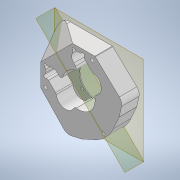
# Autodesk Inventor part: upper
Saved by Autodesk Inventor 2022 (Build 260153000, 153)
## iProperties
Created: 2022-03-17
Part Number: upper
Material: Generic
Document SubType Name: Modeling
Designer: zac-h
Density: 1 g/cm^3
Appearance: Default
Author: zac-h
Autodesk Inventor part; units mm, degrees
ref_plane "YZ Plane" through (0, 0, 0) normal (1, 0, 0) x (0, 1, 0)
ref_plane "XZ Plane" through (0, 0, 0) normal (0, 1, 0) x (-1, 0, 0)
ref_plane "XY Plane" through (0, 0, 0) normal (0, 0, 1) x (1, 0, 0)
ref_plane "Work Plane1" through (0, 0, 0) normal (0, 0, 1) x (1, 0, 0)
sketch "Sketch1" plane through (0, 0, 0) normal (0, 0, 1) x (1, 0, 0)
  line L0 (54.6745, 14.0094) -> (51.6007, 0.0667) projected
  arc A0 (54.6745, 14.0094) -> (51.7087, 23.6992) centre (44.6112, 16.228) ccw projected
  line L1 (19.1376, 54.6412) -> (51.7087, 23.6992) projected
  arc A1 (19.1376, 54.6412) -> (18.4488, 54.9162) centre (18.4488, 53.9162) ccw projected
  line L2 (-38.4967, 54.9162) -> (18.4488, 54.9162) projected
  arc A2 (-38.4967, 54.9162) -> (-54.9162, 38.4967) centre (-38.4967, 38.4967) ccw projected
  line L3 (-54.9162, -18.4488) -> (-54.9162, 38.4967) projected
  arc A3 (-54.9162, -18.4488) -> (-54.6412, -19.1376) centre (-53.9162, -18.4488) ccw projected
  line L4 (-23.6992, -51.7087) -> (-54.6412, -19.1376) projected
  arc A4 (-23.6992, -51.7087) -> (-14.0094, -54.6745) centre (-16.228, -44.6112) ccw projected
  line L5 (-0.0667, -51.6007) -> (-14.0094, -54.6745) projected
  arc A5 (-0.0667, -51.6007) -> (0.1266, -51.5369) centre (-0.282, -50.6241) ccw projected
  line L6 (17.6889, -43.6752) -> (0.1266, -51.5369) projected
  arc A6 (17.6889, -43.6752) -> (43.6752, -17.6889) centre (-3.3712, 3.3712) ccw projected
  line L7 (51.5369, -0.1266) -> (43.6752, -17.6889) projected
  arc A7 (51.5369, -0.1266) -> (51.6007, 0.0667) centre (50.6241, 0.282) ccw projected
  circle A8 centre (-3.3712, 3.3712) radius 39.37 projected
  circle A9 centre (-48.5312, 10.4312) radius 2.132 projected
  circle A10 centre (-48.5312, -2.2688) radius 2.132 projected
  circle A11 centre (-48.5312, -14.9688) radius 2.132 projected
  circle A12 centre (-10.4312, 48.5312) radius 2.132 projected
  circle A13 centre (2.2688, 48.5312) radius 2.132 projected
  circle A14 centre (14.9688, 48.5312) radius 2.132 projected
  circle A15 centre (30.3259, -30.3259) radius 2.132 projected
  circle A16 centre (-3.3712, 3.3712) radius 22.225
  line L8 (-3.3712, 3.3712) -> (14.5893, 21.3317) construction
  line L9 (-3.3712, 3.3712) -> (22.0288, 3.3712) construction
  circle A17 centre (14.5893, 21.3317) radius 2.132
  circle A18 centre (-21.3317, -14.5893) radius 2.132
  point P0 (0, 0)
  dimension "d0" = 44.45
  dimension "d1" = 25.4
  dimension "d2" = 45
  dimension "d3" = 4.264
  dimension "d6" = 360
  constraints: 4 end point, 3 centre point, 2 coincident, 1 equal length, 1 horizontal, 5 other
  measures "d0" diameter of A16
  measures "d1" distance of L8.start L8.end
  measures "d2" angle of L9 L8
  measures "d3" diameter of A17
extrude "Extrusion1" add sketch "Sketch1" along normal blind 1.2 contours L0 A7 L7 A6 L6 A5 L5 A4 L4 A3 L3 A2 L2 A1 L1 A0 | A8
sketch "Sketch2" plane through (0, 0, 1.2) normal (0, 0, 1) x (1, 0, 0)
  line L0 (18.4488, 54.9162) -> (-38.4967, 54.9162) projected
  arc A0 (-38.4967, 54.9162) -> (-54.9162, 38.4967) centre (-38.4967, 38.4967) ccw projected
  line L1 (-54.9162, 38.4967) -> (-54.9162, -18.4488) projected
  arc A1 (-54.9162, -18.4488) -> (-54.6412, -19.1376) centre (-53.9162, -18.4488) ccw projected
  line L2 (-54.6412, -19.1376) -> (-23.6992, -51.7087) projected
  arc A2 (-23.6992, -51.7087) -> (-14.0094, -54.6745) centre (-16.228, -44.6112) ccw projected
  line L3 (-14.0094, -54.6745) -> (-0.0667, -51.6007) projected
  arc A3 (-0.0667, -51.6007) -> (0.1266, -51.5369) centre (-0.282, -50.6241) ccw projected
  line L4 (0.1266, -51.5369) -> (17.6889, -43.6752) projected
  arc A4 (17.6889, -43.6752) -> (43.6752, -17.6889) centre (-3.3712, 3.3712) ccw projected
  line L5 (43.6752, -17.6889) -> (51.5369, -0.1266) projected
  arc A5 (51.5369, -0.1266) -> (51.6007, 0.0667) centre (50.6241, 0.282) ccw projected
  line L6 (51.6007, 0.0667) -> (54.6745, 14.0094) projected
  arc A6 (54.6745, 14.0094) -> (51.7087, 23.6992) centre (44.6112, 16.228) ccw projected
  line L7 (51.7087, 23.6992) -> (19.1376, 54.6412) projected
  arc A7 (19.1376, 54.6412) -> (18.4488, 54.9162) centre (18.4488, 53.9162) ccw projected
  circle A8 centre (30.3259, -30.3259) radius 2.132 projected
  circle A9 centre (14.9688, 48.5312) radius 2.132 projected
  circle A10 centre (2.2688, 48.5312) radius 2.132 projected
  circle A11 centre (-10.4312, 48.5312) radius 2.132 projected
  circle A12 centre (-48.5312, -14.9688) radius 2.132 projected
  circle A13 centre (-48.5312, -2.2688) radius 2.132 projected
  circle A14 centre (-48.5312, 10.4312) radius 2.132 projected
  circle A15 centre (-21.3317, -14.5893) radius 2.132 projected
  circle A16 centre (14.5893, 21.3317) radius 2.132 projected
  circle A17 centre (-3.3712, 3.3712) radius 22.225 projected
  circle A18 centre (14.5893, 21.3317) radius 2.132 projected
  circle A19 centre (14.5893, 21.3317) radius 12.7
  circle A20 centre (-21.3317, -14.5893) radius 12.7
  line L8 (14.5893, 21.3317) -> (-3.3712, 39.2922) construction
  line L9 (21.3245, 28.0669) -> (3.364, 46.0274)
  line L10 (-10.1064, 32.557) -> (7.8541, 14.5965)
  arc A21 (7.8541, 14.5965) -> (21.3245, 28.0669) centre (14.5893, 21.3317) ccw
  arc A22 (3.364, 46.0274) -> (-10.1064, 32.557) centre (-3.3712, 39.2922) ccw
  line L11 (14.5893, 21.3317) -> (39.9893, 21.3317) construction
  circle A23 centre (-21.3317, -14.5893) radius 2.132 projected
  line L12 (-21.3317, -14.5893) -> (-39.2922, 3.3712) construction
  line L13 (-14.5965, -7.8541) -> (-32.557, 10.1064)
  line L14 (-46.0274, -3.364) -> (-28.0669, -21.3245)
  arc A24 (-28.0669, -21.3245) -> (-14.5965, -7.8541) centre (-21.3317, -14.5893) ccw
  arc A25 (-32.557, 10.1064) -> (-46.0274, -3.364) centre (-39.2922, 3.3712) ccw
  line L15 (-21.3317, -14.5893) -> (4.0683, -14.5893) construction
  point P0 (0, 0)
  point P1 (5.6091, 30.312)
  point P2 (-30.312, -5.6091)
  point P3 (-46.6625, 9.4048)
  point P4 (-25.595, 3.1444)
  point P5 (-3.1444, 25.595)
  point P6 (-9.4048, 46.6625)
  point P7 (-8.8978, 47.0499)
  point P8 (0.1744, 48.1327)
  point P9 (2.8716, 46.4862)
  point P10 (15.3846, 34.0068)
  point P11 (18.096, 9.1254)
  point P12 (-9.1254, -18.096)
  point P13 (-34.0068, -15.3846)
  point P14 (-46.4862, -2.8716)
  point P15 (-48.1327, -0.1744)
  point P16 (-47.0499, 8.8978)
  dimension "d10" = 25.4
  dimension "d11" = 25.4
  dimension "d12" = 135
  dimension "d13" = 19.05
  dimension "d14" = 25.4
  dimension "d15" = 135
  constraints: 20 end point, 8 point on circle, 8 tangent, 6 centre point, 2 coincident, 2 equal length, 2 equal radius, 2 horizontal, 2 midpoint, 2 parallel
  measures "d10" diameter of A19
  measures "d11" distance of L8.start L8.end
  measures "d12" angle of L11 L8
  measures "d13" diameter of A22
  measures "d14" distance of L12.start L12.end
  measures "d15" angle of L15 L12
extrude "Extrusion2" add sketch "Sketch2" along normal blind 22.606 contours A7 L7 A6 L6 A5 L5 A4 L4 A3 L3 A2 L2 A1 L1 A0 L0
fillet "Fillet1" radius 3.175 14 edges at (0.1744, 48.1327, 12.503) (2.8716, 46.4862, 12.503) (-3.1444, 25.595, 12.503) (15.3846, 34.0068, 12.503) (18.096, 9.1254, 12.503) (-9.1254, -18.096, 12.503) (-34.0068, -15.3846, 12.503) (-46.4862, -2.8716, 12.503) (-48.1327, -0.1744, 12.503) (-25.595, 3.1444, 12.503) (-9.4048, 46.6625, 12.503) (-8.8978, 47.0499, 12.503) (-47.0499, 8.8978, 12.503) (-46.6625, 9.4048, 12.503)
ref_plane "Work Plane2" through (-1455.9157, 1455.9157, 0) normal (-0.7071068, -0.7071068, 0) x (0, 0, 1)
sketch "Sketch3" plane through (-1455.9157, 1455.9157, 0) normal (-0.7071068, -0.7071068, 0) x (0, 0, 1)
  line L0 (0, -1992.9228) -> (0, -1988.1137) projected
  line L1 (0, -1988.1137) -> (23.806, -2011.9197)
  line L2 (23.806, -1992.9228) -> (23.806, -2033.1894) projected
  line L3 (0, -1988.1137) -> (33.6668, -1988.1137) construction
  line L4 (23.806, -2011.9197) -> (23.806, -1988.1137)
  line L5 (23.806, -2015.151) -> (0, -2015.151) projected
  line L6 (23.806, -1988.1137) -> (0, -1988.1137)
  line L7 (0, -1988.1137) -> (23.806, -1988.1137) projected
  point P0 (0, -2058.9757)
  dimension "d19" = 45
  constraints: 8 end point, 1 collinear, 1 equal length, 1 horizontal, 1 perpendicular, 1 point on line
  measures "d19" angle of L1 L3
extrude "Extrusion3" cut sketch "Sketch3" along normal through all both and the other way through all
body "Solid1"
